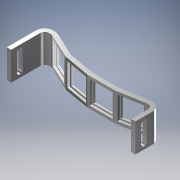
# Autodesk Inventor part: key_holder_metal
Saved by Autodesk Inventor 2018 (Build 220112000, 112)
## iProperties
Created: 2018-04-04
Part Number: key_holder_metal
Material: アルミニウム 6061
Document SubType Name: Sheet Metal
Designer: NaMACHAN
Density: 2.7 g/cm^3
Sheet Metal Rule: Default_mm
Appearance: アルミニウム - フラット
Mass: 6.46479 g
Surface Area: 40.6835 cm^2
Volume: 2.39437 cm^3
Flat Pattern Width: 2 cm
Flat Pattern Length: 12.6207 cm
Flat Pattern Area: 25.2415 cm^2
Sheet Metal Width: 20.000 mm
Sheet Metal Length: 126.207 mm
Sheet Metal Area: 2524.148 mm^2
Author: NaMACHAN
Autodesk Inventor part; units mm, degrees
ref_plane "YZ Plane" through (0, 0, 0) normal (1, 0, 0) x (0, 1, 0)
ref_plane "XZ Plane" through (0, 0, 0) normal (0, 1, 0) x (-1, 0, 0)
ref_plane "XY Plane" through (0, 0, 0) normal (0, 0, 1) x (1, 0, 0)
sketch "スケッチ2" plane through (0, 0, 0) normal (0, 1, 0) x (-1, 0, 0)
  line L0 (-9.5, -10) -> (9.5, -10)
  line L1 (9.5, -10) -> (9.5, 10)
  line L2 (9.5, 10) -> (-9.5, 10)
  line L3 (-9.5, 10) -> (-9.5, -10)
  line L4 (-9.5, -10) -> (9.5, 10) construction
  line L5 (9.5, -10) -> (-9.5, 10) construction
  point P0 (0, 0)
  dimension "d4" = 19
  dimension "d5" = 20
  measures "d4" distance of L2.end L1.end
  measures "d5" distance of L1.end L0.end
extrude "プレート1" add sketch "スケッチ2" along normal blind 3
sketch "スケッチ3" plane through (8.9791, 2.9544, -10) normal (0.1736482, -0.9848078, 0) x (0.9848078, 0.1736482, 0)
  line L0 (0, 20) -> (0, 0)
  line L1 (0, 0) -> (19, 0)
  line L2 (19, 0) -> (19, 20)
  line L3 (19, 20) -> (0, 20)
  constraints: 8 end point
edge flange "フランジ1" height 19 angle 10 thickness 3 bend radius 3 thickness toward (0.1736482, -0.9848078, 0) relief tear relief width 3 relief depth 1.5 edges at (9.5, 3, 0) wall of the first edge with corners at (8.9791, 2.9544, 10) (8.9791, 2.9544, -10) (27.6904, 6.2537, -10) (27.6904, 6.2537, 10)
bend "曲げ1"
corner "コーナー1"
sketch "スケッチ4" plane through (-8.9791, 2.9544, 10) normal (-0.1736482, -0.9848078, 0) x (0.9848078, -0.1736482, 0)
  line L0 (0, -20) -> (0, 0)
  line L1 (0, 0) -> (-19, 0)
  line L2 (-19, 0) -> (-19, -20)
  line L3 (-19, -20) -> (0, -20)
  constraints: 6 end point, 1 horizontal, 1 perpendicular, 1 vertical
edge flange "フランジ2" height 19 angle 10 thickness 3 bend radius 3 thickness toward (-0.1736482, -0.9848078, 0) relief tear relief width 3 relief depth 1.5 edges at (-9.5, 3, 0) wall of the first edge with corners at (-8.9791, 2.9544, -10) (-8.9791, 2.9544, 10) (-27.6904, 6.2537, 10) (-27.6904, 6.2537, -10)
bend "曲げ2"
corner "コーナー2"
sketch "スケッチ5" plane through (-26.9435, 6.0182, 10) normal (-0.4226183, -0.9063078, 0) x (0.9063078, -0.4226183, 0)
  line L0 (0, -20) -> (0, 0)
  line L1 (0, 0) -> (-19.395, 0)
  line L2 (-19.395, 0) -> (-19.395, -20)
  line L3 (-19.395, -20) -> (0, -20)
  constraints: 6 end point, 1 horizontal, 1 perpendicular, 1 vertical
edge flange "フランジ3" height 19 angle 15 thickness 3 bend radius 3 thickness toward (-0.4226183, -0.9063078, 0) relief tear relief width 3 relief depth 1.5 edges at (-27.6904, 6.2537, 0) wall of the first edge with corners at (-26.9435, 6.0182, -10) (-26.9435, 6.0182, 10) (-44.5213, 14.2149, 10) (-44.5213, 14.2149, -10)
bend "曲げ3"
corner "コーナー3"
sketch "スケッチ18" plane through (28.7323, 3.3449, -10) normal (0, 1, 0) x (1, 0, 0)
  line L0 (0, 20) -> (0, 0)
  line L1 (0, 0) -> (6.8755, 0)
  line L2 (6.8755, 0) -> (6.8755, 20)
  line L3 (6.8755, 20) -> (0, 20)
  constraints: 6 end point, 1 horizontal, 1 perpendicular, 1 vertical
edge flange "フランジ9" height 7.138 angle -10 thickness 3 bend radius 3 thickness toward (0, 1, 0) relief tear relief width 3 relief depth 1.5 edges at (27.6904, 6.2537, 0) wall of the first edge with corners at (28.7323, 3.3449, 10) (28.7323, 3.3449, -10) (35.6078, 3.3449, -10) (35.6078, 3.3449, 10)
bend "曲げ9"
corner "コーナー9"
sketch "スケッチ19" plane through (-47.057, 11.7771, 10) normal (0, 1, 0) x (1, 0, 0)
  line L0 (0, -20) -> (0, 0)
  line L1 (0, 0) -> (-7.3349, 0)
  line L2 (-7.3349, 0) -> (-7.3349, -20)
  line L3 (-7.3349, -20) -> (0, -20)
  constraints: 8 end point
edge flange "フランジ10" height 8 angle -25 thickness 3 bend radius 3 thickness toward (0, 1, 0) relief tear relief width 3 relief depth 1.5 edges at (-44.5213, 14.2149, 0) wall of the first edge with corners at (-47.057, 11.7771, -10) (-47.057, 11.7771, 10) (-54.3919, 11.7771, 10) (-54.3919, 11.7771, -10)
bend "曲げ10"
corner "コーナー10"
sketch "スケッチ20" plane through (32.6078, 6.3449, -10) normal (1, 0, 0) x (0, -1, 0)
  line L0 (0, 20) -> (0, 0)
  line L1 (0, 0) -> (18, 0)
  line L2 (18, 0) -> (18, 20)
  line L3 (18, 20) -> (0, 20)
  constraints: 6 end point, 1 horizontal, 1 perpendicular, 1 vertical
edge flange "フランジ11" height 15 angle -90 thickness 3 bend radius 3 thickness toward (1, 0, 0) relief tear relief width 3 relief depth 1.5 edges at (35.6078, 6.3449, 0) wall of the first edge with corners at (32.6078, 6.3449, 10) (32.6078, 6.3449, -10) (32.6078, -11.6551, -10) (32.6078, -11.6551, 10)
bend "曲げ11"
corner "コーナー11"
sketch "スケッチ21" plane through (-51.3919, 14.7771, 10) normal (-1, 0, 0) x (0, 1, 0)
  line L0 (0, -20) -> (0, 0)
  line L1 (0, 0) -> (-26.432, 0)
  line L2 (-26.432, 0) -> (-26.432, -20)
  line L3 (-26.432, -20) -> (0, -20)
  constraints: 6 end point, 1 horizontal, 1 perpendicular, 1 vertical
edge flange "フランジ12" height 23.432 angle -90 thickness 3 bend radius 3 thickness toward (-1, 0, 0) relief tear relief width 3 relief depth 1.5 edges at (-54.3919, 14.7771, 0) wall of the first edge with corners at (-51.3919, 14.7771, -10) (-51.3919, 14.7771, 10) (-51.3919, -11.6549, 10) (-51.3919, -11.6549, -10)
bend "曲げ12"
corner "コーナー12"
sketch "スケッチ27" plane through (10.017, 0.0912, -10) normal (0.1736482, -0.9848078, 0) x (0.9848078, 0.1736482, 0)
  line L0 (17.2375, 2) -> (1.2375, 2)
  line L1 (1.2375, 2) -> (1.2375, 18)
  line L2 (1.2375, 18) -> (17.2375, 18)
  line L3 (17.2375, 18) -> (17.2375, 2)
  line L4 (17.2375, 2) -> (1.2375, 18) construction
  line L5 (1.2375, 2) -> (17.2375, 18) construction
  line L6 (0, 20) -> (18.4751, 20) projected
  line L7 (0, 20) -> (0, 0) projected
  point P0 (-9.8806, 10)
  point P1 (9.2375, 10)
  point P2 (9.2375, 10)
  point P3 (9.2375, 20)
  point P4 (9.2375, 10)
  point P5 (0, 10)
  dimension "d200" = 16
  dimension "d201" = 16
  constraints: 12 end point, 6 midpoint, 2 parallel, 1 horizontal, 1 horizontal alignment, 1 perpendicular, 1 vertical alignment
  measures "d200" distance of L1.end L2.end
  measures "d201" distance of L0.end L1.end
sketch "スケッチ28" plane through (0, 0, 0) normal (0, -1, 0) x (1, 0, 0)
  line L0 (8, -8) -> (-8, -8)
  line L1 (-8, -8) -> (-8, 8)
  line L2 (-8, 8) -> (8, 8)
  line L3 (8, 8) -> (8, -8)
  line L4 (8, -8) -> (-8, 8) construction
  line L5 (-8, -8) -> (8, 8) construction
  line L6 (10.017, 10) -> (10.017, -10) projected
  line L7 (-8.9751, 10) -> (8.9751, 10) projected
  point P0 (0, 0)
  point P1 (0, 0)
  point P2 (0, 0)
  point P3 (10.017, 0)
  point P4 (0, 0)
  point P5 (0, 10)
  dimension "d204" = 16
  dimension "d205" = 16
  constraints: 12 end point, 6 midpoint, 2 parallel, 1 horizontal, 1 horizontal alignment, 1 perpendicular, 1 vertical alignment
  measures "d204" distance of L1.end L2.end
  measures "d205" distance of L0.end L1.end
extrude "押し出し14" cut sketch "スケッチ28" against normal blind 1.6
sketch "スケッチ29" plane through (-10.017, 0.0912, -10) normal (-0.1736482, -0.9848078, 0) x (0.9848078, -0.1736482, 0)
  line L0 (-0.8426, 2) -> (-16.8426, 2)
  line L1 (-16.8426, 2) -> (-16.8426, 18)
  line L2 (-16.8426, 18) -> (-0.8426, 18)
  line L3 (-0.8426, 18) -> (-0.8426, 2)
  line L4 (-0.8426, 2) -> (-16.8426, 18) construction
  line L5 (-16.8426, 2) -> (-0.8426, 18) construction
  line L6 (1.0419, 20) -> (1.0419, 0) projected
  line L7 (-17.6852, 20) -> (0, 20) projected
  point P0 (9.8806, 10)
  point P1 (-8.8426, 10)
  point P2 (-8.8426, 10)
  point P3 (1.0419, 10)
  point P4 (-8.8426, 10)
  point P5 (-8.8426, 20)
  dimension "d208" = 16
  dimension "d209" = 16
  constraints: 12 end point, 6 midpoint, 2 parallel, 1 horizontal, 1 horizontal alignment, 1 perpendicular, 1 vertical alignment
  measures "d208" distance of L1.end L2.end
  measures "d209" distance of L0.end L1.end
extrude "押し出し15" cut sketch "スケッチ29" against normal blind 1.6
sketch "スケッチ30" plane through (-28.9273, 3.6331, -10) normal (-0.4226183, -0.9063078, 0) x (0.9063078, -0.4226183, 0)
  line L0 (-1.3025, 2) -> (-17.3025, 2)
  line L1 (-17.3025, 2) -> (-17.3025, 18)
  line L2 (-17.3025, 18) -> (-1.3025, 18)
  line L3 (-1.3025, 18) -> (-1.3025, 2)
  line L4 (-1.3025, 2) -> (-17.3025, 18) construction
  line L5 (-17.3025, 2) -> (-1.3025, 18) construction
  line L6 (-18.605, 20) -> (0, 20) projected
  line L7 (0, 0) -> (0, 20) projected
  point P0 (27.7524, 10)
  point P1 (-9.3025, 10)
  point P2 (-9.3025, 10)
  point P3 (-9.3025, 20)
  point P4 (-9.3025, 10)
  point P5 (0, 10)
  dimension "d212" = 16
  dimension "d213" = 16
  constraints: 12 end point, 6 midpoint, 2 parallel, 1 horizontal, 1 horizontal alignment, 1 perpendicular, 1 vertical alignment
  measures "d212" distance of L1.end L2.end
  measures "d213" distance of L0.end L1.end
extrude "押し出し16" cut sketch "スケッチ30" against normal blind 1.6
extrude "押し出し17" cut sketch "スケッチ27" against normal blind 1.6
sketch "スケッチ31" plane through (9.7391, 1.6668, -10) normal (0.1736482, -0.9848078, 0) x (0.9848078, 0.1736482, 0)
  line L0 (16.2375, 3) -> (2.2375, 3)
  line L1 (2.2375, 3) -> (2.2375, 17)
  line L2 (2.2375, 17) -> (16.2375, 17)
  line L3 (16.2375, 17) -> (16.2375, 3)
  line L4 (16.2375, 3) -> (2.2375, 17) construction
  line L5 (2.2375, 3) -> (16.2375, 17) construction
  line L6 (1.2375, 18) -> (17.2375, 18) projected
  line L7 (20.2079, 20) -> (20.2079, 0) projected
  point P0 (-9.8806, 10)
  point P1 (9.2375, 10)
  point P2 (9.2375, 10)
  point P3 (9.2375, 18)
  point P4 (9.2375, 10)
  point P5 (2.2375, 10)
  point P6 (16.2375, 10)
  point P7 (20.2079, 10)
  dimension "d218" = 14
  dimension "d219" = 14
  constraints: 12 end point, 8 midpoint, 3 horizontal alignment, 2 parallel, 1 horizontal, 1 perpendicular, 1 vertical alignment
  measures "d218" distance of L1.end L2.end
  measures "d219" distance of L0.end L1.end
extrude "押し出し18" cut sketch "スケッチ31" against normal blind 1.4
sketch "スケッチ32" plane through (0, 1.6, 0) normal (0, -1, 0) x (1, 0, 0)
  line L0 (7, -7) -> (-7, -7)
  line L1 (-7, -7) -> (-7, 7)
  line L2 (-7, 7) -> (7, 7)
  line L3 (7, 7) -> (7, -7)
  line L4 (7, -7) -> (-7, 7) construction
  line L5 (-7, -7) -> (7, 7) construction
  line L6 (8.9751, -10) -> (8.9751, 10) projected
  line L7 (-8, 8) -> (8, 8) projected
  point P0 (0, 0)
  point P1 (0, 0)
  point P2 (0, 0)
  point P3 (8.9751, 0)
  point P4 (0, 0)
  point P5 (0, 8)
  dimension "d222" = 14
  dimension "d223" = 14
  constraints: 12 end point, 6 midpoint, 2 parallel, 1 horizontal, 1 horizontal alignment, 1 perpendicular, 1 vertical alignment
  measures "d222" distance of L1.end L2.end
  measures "d223" distance of L0.end L1.end
extrude "押し出し19" cut sketch "スケッチ32" against normal blind 1.4
sketch "スケッチ33" plane through (-9.7391, 1.6668, -10) normal (-0.1736482, -0.9848078, 0) x (0.9848078, -0.1736482, 0)
  line L0 (-1.8426, 3) -> (-15.8426, 3)
  line L1 (-15.8426, 3) -> (-15.8426, 17)
  line L2 (-15.8426, 17) -> (-1.8426, 17)
  line L3 (-1.8426, 17) -> (-1.8426, 3)
  line L4 (-1.8426, 3) -> (-15.8426, 17) construction
  line L5 (-15.8426, 3) -> (-1.8426, 17) construction
  line L6 (1.0419, 20) -> (1.0419, 0) projected
  line L7 (-16.8426, 18) -> (-0.8426, 18) projected
  point P0 (9.8806, 10)
  point P1 (-8.8426, 10)
  point P2 (-8.8426, 10)
  point P3 (1.0419, 10)
  point P4 (-8.8426, 10)
  point P5 (-8.8426, 18)
  dimension "d226" = 14
  dimension "d227" = 14
  constraints: 12 end point, 6 midpoint, 2 parallel, 1 horizontal, 1 horizontal alignment, 1 perpendicular, 1 vertical alignment
  measures "d226" distance of L1.end L2.end
  measures "d227" distance of L0.end L1.end
extrude "押し出し20" cut sketch "スケッチ33" against normal blind 1.4
sketch "スケッチ34" plane through (-28.2511, 5.0832, -10) normal (-0.4226183, -0.9063078, 0) x (0.9063078, -0.4226183, 0)
  line L0 (-2.3025, 3) -> (-16.3025, 3)
  line L1 (-16.3025, 3) -> (-16.3025, 17)
  line L2 (-16.3025, 17) -> (-2.3025, 17)
  line L3 (-2.3025, 17) -> (-2.3025, 3)
  line L4 (-2.3025, 3) -> (-16.3025, 17) construction
  line L5 (-16.3025, 3) -> (-2.3025, 17) construction
  line L6 (-17.3025, 18) -> (-1.3025, 18) projected
  line L7 (-1.3025, 18) -> (-1.3025, 2) projected
  point P0 (27.7524, 10)
  point P1 (-9.3025, 10)
  point P2 (-9.3025, 10)
  point P3 (-9.3025, 18)
  point P4 (-9.3025, 10)
  point P5 (-1.3025, 10)
  dimension "d230" = 14
  dimension "d231" = 14
  constraints: 12 end point, 6 midpoint, 2 parallel, 1 horizontal, 1 horizontal alignment, 1 perpendicular, 1 vertical alignment
  measures "d230" distance of L1.end L2.end
  measures "d231" distance of L0.end L1.end
extrude "押し出し21" cut sketch "スケッチ34" against normal blind 1.4
sketch "スケッチ35" plane through (35.6078, -11.6551, 10) normal (1, 0, 0) x (0, 0, -1)
  line L0 (4, 8) -> (16, 8)
  arc A0 (16, 4) -> (16, 8) centre (16, 6) ccw
  line L1 (16, 4) -> (4, 4)
  arc A1 (4, 8) -> (4, 4) centre (4, 6) ccw
  line L2 (20, 12) -> (20, 0) projected
  line L3 (0, 12) -> (0, 0) projected
  line L4 (0, 0) -> (20, 0) projected
  point P0 (10, 11.6551)
  dimension "d234" = 2
  dimension "d235" = 4
  dimension "d236" = 4
  dimension "d237" = 6
  constraints: 4 end point, 4 point on circle, 4 tangent, 2 centre point, 1 horizontal, 1 parallel
  measures "d234" radius of A0
  measures "d235" distance from line of L2 A0.centre
  measures "d236" distance from line of L3 A1.centre
  measures "d237" distance from line of L4 A1.centre
extrude "押し出し22" cut sketch "スケッチ35" against normal blind 100
equation "\"d6\" = Thickness"
equation "\"d7\" = BendReliefWidth"
equation "\"d8\" = BendReliefDepth"
equation "\"d9\" = MinimumRemnant"
equation "\"d10\" = TransitionRadius"
equation "\"d13\" = BendRadius"
equation "\"d14\" = CornerReliefSize"
equation "\"d15\" = GapSize"
equation "\"d16\" = JacobiRadiusSize"
equation "\"d17\" = BendReliefWidth"
equation "\"d18\" = BendReliefDepth"
equation "\"d19\" = MinimumRemnant"
equation "\"d20\" = TransitionRadius"
equation "\"d23\" = BendRadius"
equation "\"d24\" = CornerReliefSize"
equation "\"d25\" = GapSize"
equation "\"d26\" = JacobiRadiusSize"
equation "\"d27\" = BendReliefWidth"
equation "\"d28\" = BendReliefDepth"
equation "\"d29\" = MinimumRemnant"
equation "\"d30\" = TransitionRadius"
equation "\"d33\" = BendRadius"
equation "\"d34\" = CornerReliefSize"
equation "\"d35\" = GapSize"
equation "\"d36\" = JacobiRadiusSize"
equation "\"d133\" = BendReliefWidth"
equation "\"d134\" = BendReliefDepth"
equation "\"d135\" = MinimumRemnant"
equation "\"d136\" = TransitionRadius"
equation "\"d139\" = BendRadius"
equation "\"d140\" = CornerReliefSize"
equation "\"d141\" = GapSize"
equation "\"d142\" = JacobiRadiusSize"
equation "\"d143\" = BendReliefWidth"
equation "\"d144\" = BendReliefDepth"
equation "\"d145\" = MinimumRemnant"
equation "\"d146\" = TransitionRadius"
equation "\"d149\" = BendRadius"
equation "\"d150\" = CornerReliefSize"
equation "\"d151\" = GapSize"
equation "\"d152\" = JacobiRadiusSize"
equation "\"d153\" = BendReliefWidth"
equation "\"d154\" = BendReliefDepth"
equation "\"d155\" = MinimumRemnant"
equation "\"d156\" = TransitionRadius"
equation "\"d159\" = BendRadius"
equation "\"d160\" = CornerReliefSize"
equation "\"d161\" = GapSize"
equation "\"d162\" = JacobiRadiusSize"
equation "\"d163\" = BendReliefWidth"
equation "\"d164\" = BendReliefDepth"
equation "\"d165\" = MinimumRemnant"
equation "\"d166\" = TransitionRadius"
equation "\"d169\" = BendRadius"
equation "\"d170\" = CornerReliefSize"
equation "\"d171\" = GapSize"
equation "\"d172\" = JacobiRadiusSize"
equation "\"BendRadius\" = Thickness"
equation "\"BendReliefWidth\" = Thickness"
equation "\"BendReliefDepth\" = 0.5 * Thickness"
equation "\"CornerReliefSize\" = 4 * Thickness"
equation "\"MinimumRemnant\" = 2 * Thickness"
equation "\"TransitionRadius\" = BendRadius"
equation "\"JacobiRadiusSize\" = BendRadius"
equation "\"GapSize\" = Thickness"
equation "\"Thickness\" = 3"
